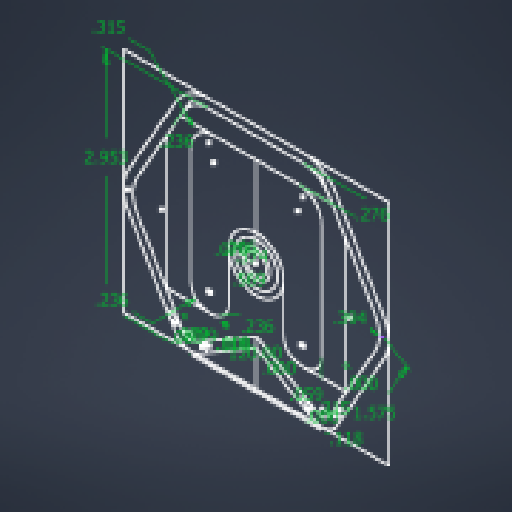
# Autodesk Inventor part: CalibrationBlockV3
Saved by Autodesk Inventor 2023 (Build 270158000, 158)
## iProperties
Created: 2022-12-27
Part Number: CalibrationBlockV3
Material: Generic
Document SubType Name: Modeling
Designer: jevan
Density: 1 g/cm^3
Appearance: Default
Author: jevan
Autodesk Inventor part; units mm, degrees
ref_plane "YZ Plane" through (0, 0, 0) normal (1, 0, 0) x (0, 1, 0)
ref_plane "XZ Plane" through (0, 0, 0) normal (0, 1, 0) x (-1, 0, 0)
ref_plane "XY Plane" through (0, 0, 0) normal (0, 0, 1) x (1, 0, 0)
sketch "Sketch1" plane through (0, 0, 0) normal (0, 0, 1) x (1, 0, 0)
  line L0 (-27.3013, -27.7128) -> (-40.4145, -5)
  line L1 (-40.4145, 5) -> (-24.5374, 32.5)
  line L2 (-15.8771, 37.5) -> (15.8771, 37.5)
  line L3 (24.5374, 32.5) -> (40.4145, 5)
  line L4 (40.4145, -5) -> (27.3013, -27.7128)
  line L5 (21.6506, -37.5) -> (-21.6506, -37.5)
  line L6 (16.3731, -30.641) -> (0, -21.188)
  line L7 (0, -21.188) -> (-16.3731, -30.641)
  circle A0 centre (0, 0) radius 4.75
  line L8 (43.3013, 0) -> (41.7543, 0)
  arc A1 (20.7032, -33.141) -> (24.8013, -32.0429) centre (22.2032, -30.5429) ccw
  arc A2 (-24.8013, -32.0429) -> (-20.7032, -33.141) centre (-22.2032, -30.5429) ccw
  arc A3 (40.4145, -5) -> (40.4145, 5) centre (31.7543, 0) ccw
  arc A4 (24.5374, 32.5) -> (15.8771, 37.5) centre (15.8771, 27.5) ccw
  arc A5 (-15.8771, 37.5) -> (-24.5374, 32.5) centre (-15.8771, 27.5) ccw
  arc A6 (-40.4145, 5) -> (-40.4145, -5) centre (-31.7543, 0) ccw
  circle A7 centre (0, 0) radius 3.375
  line L9 (0, -21.188) -> (0, -37.5)
  circle A8 centre (0, 0) radius 7.225
  line L10 (0, 0) -> (-7.225, 0)
  line L11 (-9.225, 0) -> (-9.225, -16.1218)
  line L12 (-19.2032, -35.7391) -> (0, -24.6521)
  line L13 (0, -24.6521) -> (19.2032, -35.7391)
  arc A9 (19.2032, -35.7391) -> (27.3993, -33.5429) centre (22.2032, -30.5429) ccw
  line L14 (27.3993, -33.5429) -> (43.0126, -6.5)
  arc A10 (43.0126, -6.5) -> (43.0126, 6.5) centre (31.7543, 0) ccw
  line L15 (43.0126, 6.5) -> (27.1355, 34)
  arc A11 (27.1355, 34) -> (15.8771, 40.5) centre (15.8771, 27.5) ccw
  line L16 (15.8771, 40.5) -> (-15.8771, 40.5)
  arc A12 (-15.8771, 40.5) -> (-27.1355, 34) centre (-15.8771, 27.5) ccw
  line L17 (-27.1355, 34) -> (-43.0126, 6.5)
  arc A13 (-43.0126, 6.5) -> (-43.0126, -6.5) centre (-31.7543, 0) ccw
  line L18 (-43.0126, -6.5) -> (-27.3993, -33.5429)
  arc A14 (-27.3993, -33.5429) -> (-19.2032, -35.7391) centre (-22.2032, -30.5429) ccw
  line L19 (-15.225, -22.1218) -> (-16.1451, -22.1218)
  line L20 (-22.1451, -16.1218) -> (-22.1451, 22.5)
  line L21 (-14.1451, 30.5) -> (0, 30.5)
  arc A15 (-14.1451, 30.5) -> (-22.1451, 22.5) centre (-14.1451, 22.5) ccw
  arc A16 (-22.1451, -16.1218) -> (-16.1451, -22.1218) centre (-16.1451, -16.1218) ccw
  arc A17 (-15.225, -22.1218) -> (-9.225, -16.1218) centre (-15.225, -16.1218) ccw
  line L22 (0, 0) -> (0, 30.5)
  line L23 (9.225, 0) -> (9.225, -16.1218)
  arc A18 (9.225, -16.1218) -> (15.225, -22.1218) centre (15.225, -16.1218) ccw
  line L24 (15.225, -22.1218) -> (16.1451, -22.1218)
  arc A19 (16.1451, -22.1218) -> (22.1451, -16.1218) centre (16.1451, -16.1218) ccw
  line L25 (22.1451, -16.1218) -> (22.1451, 22.5)
  arc A20 (22.1451, 22.5) -> (14.1451, 30.5) centre (14.1451, 22.5) ccw
  line L26 (14.1451, 30.5) -> (0, 30.5)
  circle A21 centre (0, 0) radius 9.225
  line L27 (-22.2032, -30.5429) -> (-24.8013, -32.0429)
  line L28 (-22.2032, -30.5429) -> (-20.7032, -33.141)
  line L29 (22.2032, -30.5429) -> (20.7032, -33.141)
  line L30 (22.2032, -30.5429) -> (24.8013, -32.0429)
  arc A22 (-25.8013, -30.3109) -> (-28.3993, -31.8109) centre (-27.1003, -31.0609) ccw
  arc A23 (-17.4711, -34.7391) -> (-18.9711, -32.141) centre (-18.2211, -33.4401) ccw
  arc A24 (28.3993, -31.8109) -> (25.8013, -30.3109) centre (27.1003, -31.0609) ccw
  arc A25 (18.9711, -32.141) -> (17.4711, -34.7391) centre (18.2211, -33.4401) ccw
  line L31 (-14.1451, 30.5) -> (-25.6921, 30.5)
  line L32 (14.1451, 30.5) -> (25.6921, 30.5)
  line L33 (-16.1451, -22.1218) -> (-30.5293, -22.1218)
  line L34 (16.1451, -22.1218) -> (30.5293, -22.1218)
  line L35 (24.8013, -32.0429) -> (40.4145, -5)
  arc A26 (40.4145, -5) -> (40.4145, 5) centre (31.7543, 0) ccw
  line L36 (40.4145, 5) -> (24.5374, 32.5)
  arc A27 (24.5374, 32.5) -> (15.8771, 37.5) centre (15.8771, 27.5) ccw
  line L37 (15.8771, 37.5) -> (-15.8771, 37.5)
  arc A28 (-15.8771, 37.5) -> (-24.5374, 32.5) centre (-15.8771, 27.5) ccw
  line L38 (-24.5374, 32.5) -> (-40.4145, 5)
  arc A29 (-40.4145, 5) -> (-40.4145, -5) centre (-31.7543, 0) ccw
  line L39 (-40.4145, -5) -> (-24.8013, -32.0429)
  arc A30 (20.7032, -33.141) -> (24.8013, -32.0429) centre (22.2032, -30.5429) ccw
  line L40 (20.7032, -33.141) -> (0, -21.188)
  line L41 (0, -21.188) -> (-20.7032, -33.141)
  arc A31 (-24.8013, -32.0429) -> (-20.7032, -33.141) centre (-22.2032, -30.5429) ccw
  line L42 (27.8503, -29.7619) -> (27.8503, -29.7619)
  line L43 (16.9221, -32.6901) -> (16.9221, -32.6901)
  line L44 (-16.9221, -32.6901) -> (-16.9221, -32.6901)
  line L45 (-27.8503, -29.7619) -> (-27.8503, -29.7619)
  arc A32 (27.3013, -27.7128) -> (27.8503, -29.7619) centre (28.6003, -28.4628) ccw
  arc A33 (16.9221, -32.6901) -> (16.3731, -30.641) centre (15.6231, -31.9401) ccw
  arc A34 (-16.3731, -30.641) -> (-16.9221, -32.6901) centre (-15.6231, -31.9401) ccw
  arc A35 (-27.8503, -29.7619) -> (-27.3013, -27.7128) centre (-28.6003, -28.4628) ccw
  line L46 (-24.5374, 32.5) -> (-21.6506, 37.5)
  line L47 (-15.8771, 37.5) -> (-21.6506, 37.5)
  line L48 (15.8771, 37.5) -> (21.6506, 37.5)
  line L49 (24.5374, 32.5) -> (21.6506, 37.5)
  line L50 (30.1451, -22.7872) -> (30.1451, 22.7872)
  line L51 (-30.1451, -22.7872) -> (-30.1451, 22.7872)
  line L52 (-44.7543, 40.5) -> (44.7543, 40.5)
  line L53 (44.7543, 40.5) -> (44.7543, -36.5429)
  line L54 (44.7543, -36.5429) -> (-44.7543, -36.5429)
  line L55 (-44.7543, -36.5429) -> (-44.7543, 40.5)
  line L56 (-3.375, 6.3883) -> (-3.375, -6.3883)
  line L57 (3.375, 6.3883) -> (3.375, -6.3883)
  line L58 (-6.3883, 3.375) -> (6.3883, 3.375)
  line L59 (-6.3883, -3.375) -> (6.3883, -3.375)
  point P0 (-43.3013, 0)
  point P1 (36.8061, -2.25)
  point P2 (6.0982, -2.25)
  point P3 (19.9965, -30.1349)
  point P4 (4.9976, -4.1562)
  point P5 (-6.0982, 2.25)
  point P6 (-36.8061, 2.25)
  point P7 (-36.8061, -2.25)
  point P8 (-6.0982, -2.25)
  point P9 (-20.3516, 30.75)
  point P10 (-4.9976, 4.1562)
  point P11 (-1.1005, 6.4062)
  point P12 (-16.4545, 33)
  point P13 (16.4545, 33)
  point P14 (1.1005, 6.4062)
  point P15 (4.9976, 4.1562)
  point P16 (20.3516, 30.75)
  point P17 (36.8061, 2.25)
  point P18 (6.0982, 2.25)
  point P19 (1.1005, -6.4062)
  point P20 (12.2023, -25.6349)
  point P21 (-4.9976, -4.1562)
  point P22 (-19.9965, -30.1349)
  point P23 (-12.2023, -25.6349)
  point P24 (-1.1005, -6.4062)
  point P25 (-9.225, -26.5141)
  point P26 (7, 0)
  point P27 (0, 7.225)
  point P28 (17.4711, -34.7391)
  point P29 (28.3993, -31.8109)
  point P30 (25.8013, -30.3109)
  point P31 (24.8013, -32.0429)
  point P32 (20.7032, -33.141)
  point P33 (18.9711, -32.141)
  point P34 (-20.7032, -33.141)
  point P35 (-24.8013, -32.0429)
  point P36 (30.1451, -22.1218)
  point P37 (30.1451, 22.7872)
  point P38 (-30.1451, 22.7872)
  point P39 (-30.1451, -22.1218)
  point P40 (-27.8503, -29.7619)
  point P41 (-16.9221, -32.6901)
  point P42 (27.8503, -29.7619)
  point P43 (15.8771, 40.5)
  point P44 (27.3013, -27.7128)
  point P45 (3.375, 3.375)
  point P46 (-3.375, 3.375)
  point P47 (-3.375, -3.375)
  point P48 (3.375, -3.375)
  dimension "d11" = 14.45
  dimension "d0" = 9.5
  dimension "d1" = 120
  dimension "d2" = 75
  dimension "d3" = 40
  dimension "d4" = 3
  dimension "d5" = 10
  dimension "d6" = 6.75
  dimension "d7" = 3
  dimension "d8" = 8
  dimension "d9" = 6
  dimension "d10" = 6
  dimension "d12" = 2
  dimension "d13" = 2
  dimension "d14" = 2
  dimension "d15" = 6
  dimension "d16" = 0
  dimension "d17" = 0
  dimension "d18" = 0
  dimension "d19" = 0
  dimension "d20" = 0
  dimension "d21" = 1.5
  dimension "d22" = 7
  dimension "d23" = 8
  constraints: 120 end point, 71 point on circle, 41 tangent, 35 centre point, 30 point on line, 17 symmetric about line, 15 perpendicular, 8 equal radius, 5 horizontal, 5 parallel, 4 coincident, 4 vertical, 2 collinear, 1 concentric, 1 midpoint, 44 other
  measures "d0" diameter of A0
  measures "d1" angle of L7 L6
  measures "d2" distance between parallel lines of L5 L2
  measures "d3" distance from line of L8.start L6
  measures "d4" radius of A1
  measures "d5" radius of A3
  measures "d6" diameter of A7
  measures "d7" distance between parallel lines of L7 L12
  measures "d8" radius of A15
  measures "d9" radius of A16
  measures "d10" distance edge to line of A17 L7
  measures "d13" distance from line of A22.centre L27
  measures "d14" distance from line of L28 A23.centre
  measures "d15" distance edge to line of A15 L1
  measures "d16" distance between parallel lines of L4 L35
  measures "d17" radial gap between concentric circles of A1 A30
  measures "d18" distance between parallel lines of L6 L40
  measures "d19" distance between parallel lines of L7 L41
  measures "d20" radial gap between concentric circles of A2 A31
  measures "d21" radius of A32
  measures "d22" distance between parallel lines of L2 L26
  measures "d23" distance between parallel lines of L25 L50
extrude "Extrusion1" add sketch "Sketch1" along normal blind 5 contours A35 A22 L18 A13 L17 A12 L16 A11 L15 A10 L14 A24 A32 L4 A3 L3 L49 L48 L2 L47 L46 L1 A6 L0 | L0 L51 L33 L19 A17 L11 A21 L23 A18 L24 L34 L50 L4 L35 L30 L29 L40 L6 L7 L41 L28 L27 L39 | L39 A22 A35 | L0 L33 L51 | L39 A2 L41 A23 L12 A14 L18 A22 | L0 A6 L1 L51 L33 | L51 L1 L31 A15 L20 A16 L33 | L27 L28 A2 | L18 A14 L54 L55 A13 | A16 L20 A15 L21 L22 A21 L11 A17 L19 | L1 A5 L2 A4 L3 L32 L26 L21 L31 | L41 A34 A23 | L55 L52 A12 L17 A13 | A14 L12 L9 L54 | L46 L47 A5 | A34 L7 L9 L12 A23 | L9 L13 A9 L54 | A8 L57 L58 A0 L22 | L22 A0 L58 L56 A8 | A21 | L26 A20 L25 A19 L24 A18 L23 A21 L22 | L6 A33 A25 L13 L9 | A9 L13 A25 L40 A1 L35 A24 L14 | A9 L14 A10 L53 L54 | L48 L49 A4 | L32 L3 L50 L34 A19 L25 A20 | L40 A25 A33 | L52 L53 A10 L15 A11 | A8 L58 L57 | L56 L58 A8 | L22 L58 A0 | A0 L58 L22 | L3 A3 L4 L34 L50 | L29 L30 A1 | A24 L35 A32 | A8 L59 L57 A0 L58 | L57 A0 L58 | L58 L56 A0 L10 A8 | L58 A0 L56 | A0 L57 A7 L58 | L58 A7 L56 A0 | L22 L10 A7 | A7 L10 L22 | L34 L4 L50 | A0 L57 | L10 A0 L56 L59 A8 | L56 L10 A0 | L57 A0 L59 A7 | L56 A0 L10 | A7 L59 A0 L56 | A8 L57 L59 | L59 L56 A8 | L59 A0 | L57 L59 A0 | A0 L59 L56 | A8 L56 L59 A0 L57
extrude "Extrusion2" add sketch "Sketch1" against normal blind 4 contours A35 A22 L18 A13 L17 A12 L16 A11 L15 A10 L14 A24 A32 L4 A3 L3 L49 L48 L2 L47 L46 L1 A6 L0 | L39 A22 A35 | L39 A2 L41 A23 L12 A14 L18 A22 | L18 A14 L54 L55 A13 | L41 A34 A23 | L55 L52 A12 L17 A13 | A14 L12 L9 L54 | L46 L47 A5 | A34 L7 L9 L12 A23 | L9 L13 A9 L54 | L6 A33 A25 L13 L9 | A9 L13 A25 L40 A1 L35 A24 L14 | A9 L14 A10 L53 L54 | L48 L49 A4 | L40 A25 A33 | L52 L53 A10 L15 A11 | A24 L35 A32
extrude "Extrusion3" cut sketch "Sketch1" along normal through all contours A8 L57 L58 A0 L22 | L22 A0 L58 L56 A8 | A8 L58 L57 | L56 L58 A8 | L22 L58 A0 | A0 L58 L22 | A8 L59 L57 A0 L58 | L57 A0 L58 | L58 L56 A0 L10 A8 | L58 A0 L56 | A0 L57 A7 L58 | L58 A7 L56 A0 | L22 L10 A7 | A7 L10 L22 | A0 L57 | L10 A0 L56 L59 A8 | L56 L10 A0 | L57 A0 L59 A7 | L56 A0 L10 | A7 L59 A0 L56 | A8 L57 L59 | L59 L56 A8 | L59 A0 | L57 L59 A0 | A0 L59 L56 | A8 L56 L59 A0 L57
extrude "Extrusion5" add sketch "Sketch1" along normal blind 0.35 contours A8 L58 L57 | L56 L58 A8 | A8 L59 L57 A0 L58 | L58 L56 A0 L10 A8 | A0 L57 | L10 A0 L56 L59 A8 | L56 L10 A0 | L56 A0 L10 | A8 L57 L59 | L59 L56 A8
extrude "Extrusion6" add sketch "Sketch1" along normal blind 0.1 contours A8 L57 L58 A0 L22 | L22 A0 L58 L56 A8 | L22 L58 A0 | A0 L58 L22 | L59 A0 | A8 L56 L59 A0 L57
body "Solid1"
